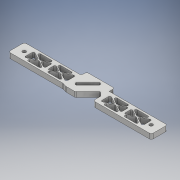
# Autodesk Inventor part: gyromount
Saved by Autodesk Inventor 2018.3 (Build 223284000, 284)
## iProperties
Created: 2018-12-20
Part Number: gyromount
Material: 一般
Document SubType Name: Modeling
Designer: shun2
Density: 1 g/cm^3
Appearance: 既定
Author: shun2
Autodesk Inventor part; units mm, degrees
ref_plane "YZ Plane" through (0, 0, 0) normal (1, 0, 0) x (0, 1, 0)
ref_plane "XZ Plane" through (0, 0, 0) normal (0, 1, 0) x (-1, 0, 0)
ref_plane "XY Plane" through (0, 0, 0) normal (0, 0, 1) x (1, 0, 0)
sketch "スケッチ1" plane through (0, 0, 0) normal (0, 0, 1) x (1, 0, 0)
  circle A0 centre (0, 0) radius 1.7
  circle A1 centre (126.625, 0) radius 1.7
  line L0 (134.804, -5.9762) -> (134.804, 6.0238)
  line L1 (-7.821, 6.0238) -> (-7.821, -5.9762)
  arc A2 (-5.821, 8.0238) -> (-7.821, 6.0238) centre (-5.821, 6.0238) ccw
  arc A3 (-7.821, -5.9762) -> (-5.821, -7.9762) centre (-5.821, -5.9762) ccw
  arc A4 (134.804, 6.0238) -> (132.804, 8.0238) centre (132.804, 6.0238) ccw
  arc A5 (132.804, -7.9762) -> (134.804, -5.9762) centre (132.804, -5.9762) ccw
  line L2 (63.4551, -0.0131) -> (60.6266, 2.8153)
  line L3 (63.4551, -0.0131) -> (67.4551, -0.0131) construction
  line L4 (63.4551, -0.0131) -> (66.3199, -2.8046)
  line L5 (60.6266, 2.8153) -> (54.9698, -2.8415)
  line L6 (60.6266, 2.8153) -> (68.6266, 2.8153) construction
  line L7 (60.6266, 2.8153) -> (66.3034, 8.4921)
  line L8 (60.6266, 2.8153) -> (68.6548, 2.8153) construction
  line L9 (66.3199, -2.8046) -> (60.5418, -8.5828)
  line L10 (66.3199, -2.8046) -> (71.9992, 2.8747)
  line L11 (66.3199, -2.8046) -> (74.3516, -2.8046) construction
  line L12 (66.3232, 9.8858) -> (65.6371, 10.6123)
  line L13 (53.5556, -2.8414) -> (52.8485, -2.1343)
  line L14 (52.8486, -0.7201) -> (64.2031, 10.6328)
  line L15 (50.8558, 13.4563) -> (74.7634, 13.4563)
  line L16 (59.1276, -9.1686) -> (51.1476, -9.1686)
  line L17 (46.8558, 8.0238) -> (-5.821, 8.0238)
  line L18 (132.804, 8.0238) -> (76.7634, 8.0238)
  line L19 (-5.821, -7.9762) -> (46.5641, -7.9762)
  line L20 (78.7545, -7.9762) -> (132.804, -7.9762)
  line L21 (73.3903, 2.897) -> (76.1225, 0.3354)
  line L22 (48.8558, 10.0238) -> (48.8558, 11.4563)
  line L23 (76.7634, 11.4563) -> (76.7634, 8.0238)
  line L24 (76.7545, -1.1236) -> (76.7545, -5.9762)
  arc A6 (46.8558, 8.0238) -> (48.8558, 10.0238) centre (46.8558, 10.0238) ccw
  arc A7 (50.8558, 13.4563) -> (48.8558, 11.4563) centre (50.8558, 11.4563) ccw
  arc A8 (76.7634, 11.4563) -> (74.7634, 13.4563) centre (74.7634, 11.4563) ccw
  line L25 (50.5762, -9.0852) -> (47.1354, -8.0595)
  arc A9 (47.1354, -8.0595) -> (46.5641, -7.9762) centre (46.5641, -9.9762) ccw
  arc A10 (50.5762, -9.0852) -> (51.1476, -9.1686) centre (51.1476, -7.1686) ccw
  arc A11 (76.7545, -1.1236) -> (76.1225, 0.3354) centre (74.7545, -1.1236) ccw
  arc A12 (76.7545, -5.9762) -> (78.7545, -7.9762) centre (78.7545, -5.9762) ccw
  arc A13 (59.1276, -9.1686) -> (60.5418, -8.5828) centre (59.1276, -7.1686) ccw
  arc A14 (52.8486, -0.7201) -> (52.8485, -2.1343) centre (53.5557, -1.4273) ccw
  arc A15 (53.5556, -2.8414) -> (54.9698, -2.8415) centre (54.2627, -2.1344) ccw
  arc A16 (65.6371, 10.6123) -> (64.2031, 10.6328) centre (64.9101, 9.9256) ccw
  arc A17 (66.3034, 8.4921) -> (66.3232, 9.8858) centre (65.5963, 9.1992) ccw
  arc A18 (73.3903, 2.897) -> (71.9992, 2.8747) centre (72.7063, 2.1675) ccw
  arc A19 (15.9698, -0.7397) -> (14.7602, -0.7647) centre (15.3856, -1.7515) ccw
  line L26 (15.9698, -0.7397) -> (21.6953, -4.0454)
  arc A20 (21.1112, -6.2255) -> (21.6953, -4.0454) centre (21.1112, -5.0572) ccw
  line L27 (21.1112, -6.2255) -> (10.1699, -6.2255)
  arc A21 (9.5444, -4.0704) -> (10.1699, -6.2255) centre (10.1699, -5.0572) ccw
  line L28 (9.5444, -4.0704) -> (14.7602, -0.7647)
  arc A22 (22.6232, -3.4465) -> (24.325, -2.4071) centre (23.1567, -2.4071) ccw
  line L29 (22.6232, -3.4465) -> (17.9962, -1.0715)
  arc A23 (17.9949, 1.0066) -> (17.9962, -1.0715) centre (18.5297, -0.0321) ccw
  line L30 (17.9949, 1.0066) -> (22.6263, 3.3666)
  arc A24 (24.325, 2.3257) -> (22.6263, 3.3666) centre (23.1567, 2.3257) ccw
  line L31 (24.325, 2.3257) -> (24.325, -2.4071)
  arc A25 (10.1699, 6.1672) -> (9.5444, 4.0121) centre (10.1699, 4.9989) ccw
  line L32 (10.1699, 6.1672) -> (21.1112, 6.1672)
  arc A26 (21.6953, 3.9871) -> (21.1112, 6.1672) centre (21.1112, 4.9989) ccw
  line L33 (21.6953, 3.9871) -> (15.9698, 0.6815)
  arc A27 (14.7602, 0.7065) -> (15.9698, 0.6815) centre (15.3856, 1.6933) ccw
  line L34 (14.7602, 0.7065) -> (9.5444, 4.0121)
  arc A28 (6.3779, 4.3006) -> (4.6749, 3.2743) centre (5.8431, 3.2619) ccw
  line L35 (6.3779, 4.3006) -> (12.7763, 1.0066)
  arc A29 (12.775, -1.0715) -> (12.7763, 1.0066) centre (12.2415, -0.0321) ccw
  line L36 (12.775, -1.0715) -> (6.3064, -4.3918)
  arc A30 (4.6046, -3.34) -> (6.3064, -4.3918) centre (5.7729, -3.3524) ccw
  line L37 (4.6046, -3.34) -> (4.6749, 3.2743)
  arc A31 (30.2166, 6.1672) -> (29.6325, 3.9871) centre (30.2166, 4.9989) ccw
  arc A32 (28.7015, 3.3666) -> (27.0028, 2.3257) centre (28.1711, 2.3257) ccw
  arc A33 (29.6325, -4.0454) -> (30.2166, -6.2255) centre (30.2166, -5.0572) ccw
  arc A34 (27.0028, -2.4071) -> (28.7046, -3.4465) centre (28.1711, -2.4071) ccw
  line L38 (33.3328, 1.0066) -> (28.7015, 3.3666)
  arc A35 (33.3316, -1.0715) -> (33.3328, 1.0066) centre (32.7981, -0.0321) ccw
  line L39 (28.7046, -3.4465) -> (33.3316, -1.0715)
  line L40 (29.6325, 3.9871) -> (35.358, 0.6815)
  arc A36 (35.358, 0.6815) -> (36.5676, 0.7065) centre (35.9422, 1.6933) ccw
  arc A37 (36.5676, -0.7647) -> (35.358, -0.7397) centre (35.9422, -1.7515) ccw
  line L41 (35.358, -0.7397) -> (29.6325, -4.0454)
  line L42 (41.1579, 6.1672) -> (30.2166, 6.1672)
  line L43 (30.2166, -6.2255) -> (41.1579, -6.2255)
  line L44 (27.0028, 2.3257) -> (27.0028, -2.4071)
  arc A38 (38.5515, 1.0066) -> (38.5528, -1.0715) centre (39.0863, -0.0321) ccw
  line L45 (36.5676, 0.7065) -> (41.7834, 4.0121)
  line L46 (41.7834, -4.0704) -> (36.5676, -0.7647)
  arc A39 (41.7834, 4.0121) -> (41.1579, 6.1672) centre (41.1579, 4.9989) ccw
  arc A40 (41.1579, -6.2255) -> (41.7834, -4.0704) centre (41.1579, -5.0572) ccw
  line L47 (44.9499, 4.3006) -> (38.5515, 1.0066)
  line L48 (38.5528, -1.0715) -> (45.0214, -4.3918)
  line L49 (46.7232, -3.34) -> (46.6529, 3.2743)
  arc A41 (45.0214, -4.3918) -> (46.7232, -3.34) centre (45.5549, -3.3524) ccw
  arc A42 (46.6529, 3.2743) -> (44.9499, 4.3006) centre (45.4847, 3.2619) ccw
  arc A43 (97.9717, 3.9871) -> (97.3875, 6.1672) centre (97.3875, 4.9989) ccw
  arc A44 (100.6014, 2.3257) -> (98.9026, 3.3666) centre (99.4331, 2.3257) ccw
  arc A45 (97.3875, -6.2255) -> (97.9717, -4.0454) centre (97.3875, -5.0572) ccw
  arc A46 (98.8996, -3.4465) -> (100.6014, -2.4071) centre (99.4331, -2.4071) ccw
  line L50 (94.2713, 1.0066) -> (98.9026, 3.3666)
  arc A47 (94.2713, 1.0066) -> (94.2726, -1.0715) centre (94.8061, -0.0321) ccw
  line L51 (98.8996, -3.4465) -> (94.2726, -1.0715)
  line L52 (97.9717, 3.9871) -> (92.2461, 0.6815)
  arc A48 (91.0366, 0.7065) -> (92.2461, 0.6815) centre (91.662, 1.6933) ccw
  arc A49 (92.2461, -0.7397) -> (91.0366, -0.7647) centre (91.662, -1.7515) ccw
  line L53 (92.2461, -0.7397) -> (97.9717, -4.0454)
  line L54 (86.4462, 6.1672) -> (97.3875, 6.1672)
  line L55 (97.3875, -6.2255) -> (86.4462, -6.2255)
  line L56 (100.6014, 2.3257) -> (100.6014, -2.4071)
  arc A50 (89.0514, -1.0715) -> (89.0527, 1.0066) centre (88.5179, -0.0321) ccw
  line L57 (91.0366, 0.7065) -> (85.8208, 4.0121)
  line L58 (85.8208, -4.0704) -> (91.0366, -0.7647)
  arc A51 (86.4462, 6.1672) -> (85.8208, 4.0121) centre (86.4462, 4.9989) ccw
  arc A52 (85.8208, -4.0704) -> (86.4462, -6.2255) centre (86.4462, -5.0572) ccw
  line L59 (82.6542, 4.3006) -> (89.0527, 1.0066)
  line L60 (89.0514, -1.0715) -> (82.5827, -4.3918)
  line L61 (80.881, -3.34) -> (80.9512, 3.2743)
  arc A53 (80.881, -3.34) -> (82.5827, -4.3918) centre (82.0492, -3.3524) ccw
  arc A54 (82.6542, 4.3006) -> (80.9512, 3.2743) centre (82.1195, 3.2619) ccw
  arc A55 (111.6344, 0.6815) -> (112.8439, 0.7065) centre (112.2185, 1.6933) ccw
  arc A56 (112.8439, -0.7647) -> (111.6344, -0.7397) centre (112.2185, -1.7515) ccw
  line L62 (117.4343, 6.1672) -> (106.493, 6.1672)
  line L63 (106.493, -6.2255) -> (117.4343, -6.2255)
  line L64 (112.8439, 0.7065) -> (118.0597, 4.0121)
  line L65 (118.0597, -4.0704) -> (112.8439, -0.7647)
  arc A57 (117.4343, -6.2255) -> (118.0597, -4.0704) centre (117.4343, -5.0572) ccw
  arc A58 (114.8279, 1.0066) -> (114.8291, -1.0715) centre (115.3626, -0.0321) ccw
  arc A59 (109.6079, -1.0715) -> (109.6092, 1.0066) centre (109.0744, -0.0321) ccw
  line L66 (105.9088, 3.9871) -> (111.6344, 0.6815)
  line L67 (109.6092, 1.0066) -> (104.9779, 3.3666)
  line L68 (111.6344, -0.7397) -> (105.9088, -4.0454)
  line L69 (104.981, -3.4465) -> (109.6079, -1.0715)
  arc A60 (106.493, 6.1672) -> (105.9088, 3.9871) centre (106.493, 4.9989) ccw
  arc A61 (104.9779, 3.3666) -> (103.2791, 2.3257) centre (104.4475, 2.3257) ccw
  line L70 (103.2791, 2.3257) -> (103.2791, -2.4071)
  arc A62 (103.2791, -2.4071) -> (104.981, -3.4465) centre (104.4475, -2.4071) ccw
  arc A63 (105.9088, -4.0454) -> (106.493, -6.2255) centre (106.493, -5.0572) ccw
  line L71 (121.2263, 4.3006) -> (114.8279, 1.0066)
  line L72 (114.8291, -1.0715) -> (121.2978, -4.3918)
  arc A64 (122.9293, 3.2743) -> (121.2263, 4.3006) centre (121.761, 3.2619) ccw
  line L73 (122.9995, -3.34) -> (122.9293, 3.2743)
  arc A65 (121.2978, -4.3918) -> (122.9995, -3.34) centre (121.8313, -3.3524) ccw
  arc A66 (118.0597, 4.0121) -> (117.4343, 6.1672) centre (117.4343, 4.9989) ccw
  point P0 (134.804, 8.0238)
  point P1 (134.804, -7.9762)
  point P2 (-7.821, 8.0238)
  point P3 (54.2627, -3.5487)
  point P4 (66.9906, 9.1793)
  point P5 (72.6839, 3.5594)
  point P6 (64.9306, 11.3602)
  point P7 (52.1415, -1.4272)
  point P8 (59.956, -9.1686)
  point P9 (15.0236, -1.4895)
  point P10 (36.3042, -1.4895)
  point P11 (91.3, -1.4895)
  point P12 (112.5805, -1.4895)
  dimension "d0" = 3.4
  dimension "d1" = 3.4
  dimension "d2" = 126.625
  dimension "d3" = 142.625
  dimension "d4" = 16
  dimension "d5" = 2
  dimension "d6" = 2
  dimension "d19" = 4
  dimension "d20" = 135
  dimension "d21" = 4
  dimension "d22" = 9
  dimension "d23" = 135
  dimension "d24" = 9
  dimension "d25" = 45
  dimension "d26" = 9
  dimension "d27" = 9
  dimension "d28" = 45
  dimension "d29" = 3
  dimension "d30" = 3
  dimension "d31" = 2
  dimension "d33" = 1
  constraints: 148 end point, 130 point on circle, 67 centre point, 38 tangent, 15 point on line, 12 equal radius, 8 parallel, 7 horizontal, 5 perpendicular, 4 equal length, 1 coincident, 1 collinear
  measures "d0" diameter of A0
  measures "d1" diameter of A1
  measures "d2" distance of point (0, 0) A1.centre
  measures "d3" distance of point (-7.821, 8.024) point (134.804, 8.024)
  measures "d4" distance of point (134.804, 8.024) point (134.804, -7.976)
  measures "d5" radius of A2
  measures "d6" radius of A3
  measures "d19" distance of L2.start L2.end
  measures "d20" angle of L3 L2
  measures "d21" distance of L2.start L4.end
  measures "d22" distance of L2.end point (54.263, -3.549)
  measures "d23" angle of L5 L6
  measures "d24" distance of L2.end point (66.991, 9.179)
  measures "d25" angle of L8 L7
  measures "d26" distance of point (59.956, -9.169) L4.end
  measures "d27" distance of L4.end point (72.684, 3.559)
  measures "d28" angle of L11 L10
  measures "d29" distance of point (66.991, 9.179) point (64.931, 11.36)
  measures "d30" distance of point (54.263, -3.549) point (52.141, -1.427)
  measures "d31" radius of A6
  measures "d33" radius of A14
extrude "押し出し1" add sketch "スケッチ1" along normal blind 5
